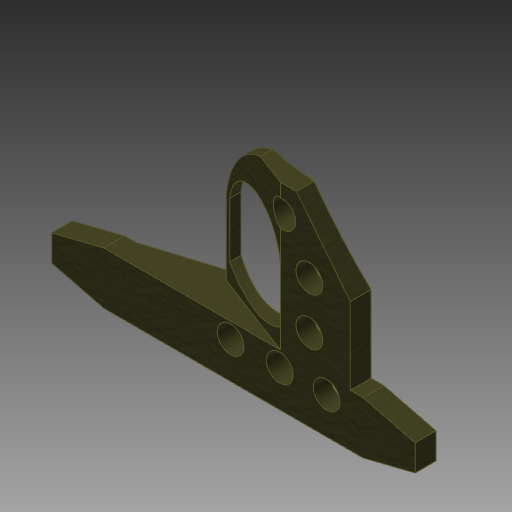
# Autodesk Inventor part: JF-JM-HC0011
Saved by Autodesk Inventor 2018.2 (Build 222227000, 227)
## iProperties
Created: 2008-12-09
Part Number: JF-JM-HC0011
Document SubType Name: Modeling
Designer: Ning-long Xu
Density: 4.43 g/cm^3
Material: TITANIUM, 6AL-4V, ANNEALED
Description: BarrelCtxPlateSlopedLeft_nx_08
Mass: 0.602365 g
Surface Area: 3.42709 cm^2
Volume: 0.133562 cm^3
Appearance: Metal-Ti
Project: COMMON
Vendor: HHMI: JRC - ID&F
ALTERED ITEM PART NUMBER: N/A
ALTERED ITEM VENDOR: N/A
SPECIAL FINISH: NONE
SURFACE ROUGHNESS: 32 Ra
LAB/DEPT: COMMON
REQUESTING SCIENTIST: COMMON
DESIGN DEPARTMENT: HHMI: JRC - ID&F
ALTERED ITEM DESCRIPTION: N/A
Author: Ning-long Xu
Revision Number: A
Autodesk Inventor part; units mm, degrees
ref_plane "YZ Plane" through (0, 0, 0) normal (1, 0, 0) x (0, 1, 0)
ref_plane "XZ Plane" through (0, 0, 0) normal (0, 1, 0) x (-1, 0, 0)
ref_plane "XY Plane" through (0, 0, 0) normal (0, 0, 1) x (1, 0, 0)
sketch "HeadplateSketch" plane through (0, 0, 0) normal (0, 0, 1) x (1, 0, 0)
  line L0 (22.2193, -2.4109) -> (25.4193, -1.6109)
  line L1 (25.4193, -1.6109) -> (25.4193, -0.0109)
  line L2 (6.3193, 0.7891) -> (3.1193, -0.0109)
  line L3 (3.1193, -1.6109) -> (3.1193, -0.0109)
  line L4 (6.3193, 0.7891) -> (22.2193, 0.7891)
  line L5 (22.2193, 0.7891) -> (25.4193, -0.0109)
  line L6 (17.1922, 9.6958) -> (17.1922, -2.4109)
  line L7 (17.1922, 9.6958) -> (18.128, 9.6958)
  line L8 (17.1922, 9.6958) -> (15.1602, 9.6958)
  line L9 (11.7996, 5.443) -> (11.7996, -2.4109)
  line L10 (21.4383, 5.5008) -> (21.4383, -2.4109)
  line L11 (21.4383, 5.5008) -> (18.128, 9.6958)
  arc A0 (15.1602, 9.6958) -> (11.7996, 5.443) centre (17.4689, 4.4173) ccw
  line L12 (3.1193, -1.6109) -> (6.3193, -2.4109)
  line L13 (6.3193, -2.4109) -> (22.2193, -2.4109)
  point P0 (11.7996, 0.7891)
  dimension "d95" = 3.2
  dimension "d102" = 1.6
  dimension "d104" = 3.2
  dimension "d106" = 0.8
  dimension "d109" = 1.6
  dimension "d110" = 3.2
  dimension "d112" = 22.3
  dimension "d113" = 15.9
  constraints: 29 end point, 5 point on line, 4 perpendicular, 3 parallel, 2 point on circle, 1 centre point, 1 horizontal
  measures "d95" horizontal distance of L2.start L2.end
  measures "d102" distance of L0.end L1.end
  measures "d104" horizontal distance of L0.start L0.end
  measures "d106" vertical distance of L1.end L4.end
  measures "d109" distance of L3.start L2.end
  measures "d110" horizontal distance of L4.end L1.end
  measures "d112" distance between parallel lines of L1 L3
  measures "d113" distance of L2.start L4.end
extrude "拉伸1" add sketch "HeadplateSketch" along normal blind 1.27
extrude "拉伸8" add sketch "HeadplateSketch" against normal blind 1.5 contours L13 L6 L4 L10 | L4 L6 L7 L11 L10 | L13 L9 L4 L6 | L4 L9 A0 L8 L6
sketch "草图2" plane through (15.1602, 9.6958, 1.27) normal (0, 1, 0) x (1, 0, 0)
  line L0 (-3.3633, 2.0352) -> (1.9994, 0)
  arc A0 (-3.3633, 2.77) -> (6.2787, 1.2693) centre (3.7754, 16.9113) ccw
  line L1 (1.9994, 0) -> (6.2787, 0)
  line L2 (-3.3633, 2.77) -> (6.2787, 2.77)
  line L3 (2.9678, 2.77) -> (0, 2.77) projected
  line L4 (6.2787, 1.2693) -> (6.2787, 2.77)
  line L5 (-3.3633, 0) -> (1.9994, 0)
  line L6 (0, 0) -> (2.9678, 0) projected
  line L7 (2.9678, 0) -> (2.9678, 2.77) projected
  line L8 (-3.3633, 0) -> (-3.3633, 2.0352)
  constraints: 12 end point, 2 point on circle, 2 point on line, 1 centre point, 1 parallel, 1 perpendicular
extrude "拉伸4" cut sketch "草图2" against normal up to next contours A0 L2 L7 | L7 L2 L4 A0
sketch "草图6" plane through (6.3193, -2.4109, 0) normal (0, -1, 0) x (1, 0, 0)
  line L0 (0, 0) -> (5.4803, 0)
  line L1 (0.6566, 0) -> (5.4803, -1.4987)
  line L2 (5.4803, 0) -> (5.4803, -1.4987)
  line L3 (0.6566, 0) -> (5.4803, 0)
  arc A0 (15.1197, 0.0007) -> (5.4803, -1.4987) centre (12.6164, -15.6413) ccw projected
  line L4 (5.4803, 0) -> (5.4803, -1.4987) projected
  dimension "d119" = 0
  dimension "d120" = 0
  constraints: 8 end point, 1 perpendicular, 1 point on line
  measures "d119" distance between parallel lines of L2 L4
  measures "d120" distance of L4.end L1.end
extrude "拉伸7" add sketch "草图6" against normal up to surface (3.2 mm away)
sketch "草图3" plane through (6.3193, 0.7891, 0) normal (0, 1, 0) x (1, 0, 0)
  line L0 (0, -1.27) -> (5.4803, -1.27) projected
  line L1 (5.4803, 0) -> (5.4803, -1.27) projected
  line L2 (5.4803, 0) -> (0, 0) projected
  line L3 (0, 0) -> (0, -1.27) projected
  line L4 (5.4803, -1.27) -> (16.1538, -1.27)
  line L5 (16.1538, -1.27) -> (17.1139, -1.27)
  line L6 (17.1139, -1.27) -> (17.1139, 0.0011)
  constraints: 6 end point, 2 perpendicular, 1 collinear
extrude "拉伸9" cut sketch "草图2" against normal up to surface (8.9067 mm away) contours L0 L5 L8
sketch "草图4" plane through (0, 0, 1.27) normal (0, 0, 1) x (1, 0, 0)
  circle A0 centre (17.2686, 8.053) radius 0.825
  circle A1 centre (18.9292, 5.5008) radius 0.825
  circle A2 centre (18.9292, 2.5892) radius 0.825
  circle A3 centre (17.1095, -0.1732) radius 0.825
  line L0 (6.3193, 0.7891) -> (11.7996, 0.7891) projected
  line L1 (12.1356, 5.3815) -> (12.1356, 2.0023)
  line L2 (12.1356, 5.3815) -> (17.1561, 5.3815)
  line L3 (17.1561, 5.3815) -> (17.1561, 2.008)
  line L4 (17.1561, 2.008) -> (12.1356, 2.008)
  line L5 (11.7983, 4.0675) -> (12.1356, 4.0675)
  arc A4 (17.1561, 5.3815) -> (12.1356, 5.3815) centre (14.6459, 4.9584) ccw
  arc A5 (12.1356, 2.008) -> (17.1561, 2.008) centre (14.6459, 5.3033) ccw
  circle A6 centre (19.9896, -0.1732) radius 0.825
  circle A7 centre (14.1001, -0.1732) radius 0.825
  point P0 (21.4383, 5.5008)
  dimension "d121" = 0.9623
  constraints: 10 end point, 8 centre point, 5 perpendicular, 4 point on circle, 3 horizontal alignment, 2 point on line, 1 vertical alignment
  measures "d121" distance from line of L0 A7.centre
extrude "拉伸10" cut sketch "草图4" against normal through all contours L2 L3 L4 L1 | A4 L2 | L4 A5
hole "打孔7" at (18.9292, 5.5008, 1.27) at (18.9292, 2.5892, 1.27) at (17.1095, -0.1732, 1.27) at (17.2686, 8.053, 1.27) direction (0, 0, -1) diameter 1.65 end through all
hole "打孔8" at (14.1001, -0.1732, 1.27) at (19.9896, -0.1732, 1.27) direction (0, 0, -1) diameter 1.65 end through all
body "Solid1"
